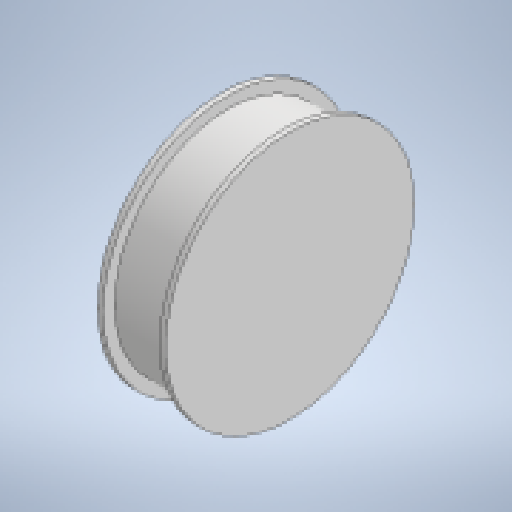
# Autodesk Inventor part: spool
Saved by Autodesk Inventor 2023 (Build 270158000, 158)
## iProperties
Created: 2022-04-19
Part Number: spool
Material: Generic
Document SubType Name: Modeling
Designer: carson
Density: 1 g/cm^3
Appearance: Default
Author: carson
Autodesk Inventor part; units mm, degrees
ref_plane "YZ Plane" through (0, 0, 0) normal (1, 0, 0) x (0, 1, 0)
ref_plane "XZ Plane" through (0, 0, 0) normal (0, 1, 0) x (-1, 0, 0)
ref_plane "XY Plane" through (0, 0, 0) normal (0, 0, 1) x (1, 0, 0)
sketch "Sketch1" plane through (0, 0, 0) normal (1, 0, 0) x (0, 1, 0)
  circle A0 centre (0, 0) radius 20
  dimension "d0" = 40
  constraints: 1 centre point, 1 coincident
  measures "d0" diameter of A0
extrude "Extrusion1" add sketch "Sketch1" along normal blind 10
sketch "Sketch2" plane through (10, 0, 0) normal (1, 0, 0) x (0, 0, -1)
  circle A0 centre (0, 0) radius 22
  dimension "d3" = 44
  constraints: 1 centre point, 1 coincident
  measures "d3" diameter of A0
extrude "Extrusion2" add sketch "Sketch2" along normal blind 1
sketch "Sketch3" plane through (0, 0, 0) normal (-1, 0, 0) x (0, 0, 1)
  circle A0 centre (0, 0) radius 22
  constraints: 1 centre point, 1 coincident
extrude "Extrusion3" add sketch "Sketch3" along normal blind 1
sketch "Sketch4" plane through (11, 0, 0) normal (1, 0, 0) x (0, 0, -1)
  circle A0 centre (0, 0) radius 2.5
  line L0 (0, 2.5) -> (0, 2.5)
  line L1 (2, -1.5) -> (-2, -1.5)
  line L2 (-2.5, 0) -> (2.5, 0)
  line L3 (2, 1.5) -> (-2, 1.5)
  dimension "d8" = 5
  dimension "d10" = 1.5
  constraints: 8 end point, 6 point on circle, 2 horizontal, 2 symmetric about line, 1 centre point, 1 coincident, 1 parallel
  measures "d8" diameter of A0
  measures "d10" distance from line of point (0, 0) L1
extrude "Extrusion4" cut sketch "Sketch4" against normal blind 12 contours L2 A0 L3 | A0 L1 L2
body "Solid1"
